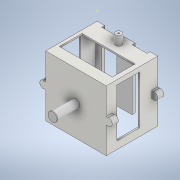
# Autodesk Inventor part: elevador_caixa_com_estabi v2
Saved by Autodesk Inventor 2021 (Build 250183000, 183)
## iProperties
Created: 2020-09-22
Part Number: elevador_caixa_com_estabi v2
Material: Genérico
Document SubType Name: Modeling
Designer: evert
Density: 1 g/cm^3
Appearance: Padrão
Author: evert
Autodesk Inventor part; units mm, degrees
ref_plane "YZ Plane" through (0, 0, 0) normal (1, 0, 0) x (0, 1, 0)
ref_plane "XZ Plane" through (0, 0, 0) normal (0, 1, 0) x (-1, 0, 0)
ref_plane "XY Plane" through (0, 0, 0) normal (0, 0, 1) x (1, 0, 0)
sketch "Esboço1" plane through (0, 0, 0) normal (0, 0, 1) x (1, 0, 0)
  line L0 (0, 0) -> (40, 0)
  line L1 (40, 0) -> (40, 40)
  line L2 (40, 40) -> (0, 40)
  line L3 (0, 40) -> (0, 0)
  dimension "d0" = 40
  dimension "d1" = 40
  constraints: 8 end point, 2 parallel, 1 horizontal, 1 perpendicular
  measures "d0" distance of L2.end L1.end
  measures "d1" distance of L0.end L1.end
extrude "Extrusão1" add sketch "Esboço1" along normal blind 2
sketch "Esboço2" plane through (0, 0, 2) normal (0, 0, 1) x (1, 0, 0)
  line L0 (0, 40) -> (0, 0) projected
  line L1 (0, 0) -> (1, 0)
  line L2 (0, 0) -> (40, 0) projected
  line L3 (0, 0) -> (0, 40)
  line L4 (40, 40) -> (0, 40) projected
  line L5 (40, 0) -> (40, 40) projected
  line L6 (40, 40) -> (40, 0)
  line L7 (40, 0) -> (39, 0)
  line L8 (39, 0) -> (39, 39)
  line L9 (39, 39) -> (1, 39)
  line L10 (1, 39) -> (1, 0)
  constraints: 14 end point, 2 collinear, 2 perpendicular, 2 point on line, 1 vertical
extrude "Extrusão2" add sketch "Esboço2" along normal blind 10 contours L4 L5 L2 L8 L9 L10 L1 L0
sketch "Esboço3" plane through (0, 0, 12) normal (0, 0, 1) x (1, 0, 0)
  line L0 (0, 40) -> (2, 40)
  line L1 (40, 40) -> (0, 40) projected
  line L2 (1, 39) -> (39, 39) projected
  line L3 (2, 39) -> (1, 39)
  line L4 (1, 39) -> (1, 38)
  line L5 (1, 0) -> (1, 39) projected
  line L6 (0, 38) -> (0, 40)
  line L7 (2, 40) -> (2, 39)
  line L8 (1, 38) -> (0, 38)
  line L9 (0, 40) -> (0, 0) projected
  constraints: 12 end point, 3 point on line, 1 collinear, 1 parallel, 1 perpendicular, 1 vertical
extrude "Extrusão3" add sketch "Esboço3" along normal blind 20
sketch "Esboço4" plane through (0, 0, 12) normal (0, 0, 1) x (1, 0, 0)
  line L0 (40, 40) -> (37, 40)
  line L1 (40, 40) -> (0, 40) projected
  line L2 (39, 39) -> (1, 39) projected
  line L3 (37, 39) -> (39, 39)
  line L4 (39, 39) -> (39, 37)
  line L5 (39, 39) -> (39, 0) projected
  line L6 (40, 0) -> (40, 40) projected
  line L7 (40, 37) -> (40, 40)
  line L8 (37, 40) -> (37, 39)
  line L9 (39, 37) -> (40, 37)
  line L10 (40, 40) -> (37, 40)
  line L11 (37, 39) -> (39, 39)
  line L12 (39, 39) -> (39, 37)
  point P0 (0, 0)
  constraints: 18 end point, 3 collinear, 2 horizontal, 2 perpendicular, 2 point on line
extrude "Extrusão4" add sketch "Esboço4" along normal blind 20
sketch "Esboço5" plane through (0, 0, 2) normal (0, 0, 1) x (1, 0, 0)
  point P0 (0, 0)
sketch "Esboço6" plane through (0, 0, 12) normal (0, 0, 1) x (1, 0, 0)
  line L0 (0, 38) -> (0, 0) projected
  line L1 (1, 0) -> (1, 38) projected
  line L2 (0, 0) -> (1, 0)
  line L3 (1, 0) -> (1, 5)
  line L4 (1, 5) -> (0, 5)
  line L5 (0, 5) -> (0, 0)
  line L6 (0, 0) -> (40, 0) projected
  line L7 (39, 0) -> (39, 39) projected
  line L8 (40, 0) -> (39, 0)
  line L9 (39, 0) -> (39, 5)
  line L10 (39, 5) -> (40, 5)
  line L11 (40, 5) -> (40, 0)
  constraints: 16 end point, 4 parallel, 3 point on line, 2 horizontal, 2 perpendicular
extrude "Extrusão5" add sketch "Esboço6" along normal blind 20
sketch "Esboço7" plane through (0, 0, 32) normal (0, 0, 1) x (1, 0, 0)
  line L0 (0, 38) -> (0, 5) projected
  line L1 (0, 38) -> (1, 38)
  line L2 (1, 5) -> (1, 38) projected
  line L3 (1, 38) -> (1, 5)
  line L4 (1, 5) -> (0, 5)
  line L5 (0, 40) -> (0, 38) projected
  line L6 (0, 5) -> (0, 38)
  point P0 (0, 0)
  constraints: 8 end point, 2 perpendicular, 1 collinear, 1 horizontal
extrude "Extrusão6" add sketch "Esboço7" against normal blind 5
sketch "Esboço8" plane through (0, 0, 32) normal (0, 0, 1) x (1, 0, 0)
  line L0 (2, 40) -> (0, 40) projected
  line L1 (39, 39) -> (1, 39) projected
  line L2 (2, 40) -> (37, 40)
  line L3 (37, 40) -> (37, 39)
  line L4 (37, 39) -> (2, 39)
  line L5 (2, 39) -> (2, 40)
  point P0 (0, 0)
  constraints: 8 end point, 2 parallel, 1 horizontal, 1 perpendicular, 1 point on line
extrude "Extrusão7" add sketch "Esboço8" against normal blind 5
sketch "Esboço9" plane through (0, 0, 32) normal (0, 0, 1) x (1, 0, 0)
  line L0 (40, 0) -> (40, 40) projected
  line L1 (39, 37) -> (40, 37)
  line L2 (40, 37) -> (40, 5)
  line L3 (40, 5) -> (39, 5)
  line L4 (39, 5) -> (39, 37)
  point P0 (0, 0)
  constraints: 8 end point, 2 parallel, 1 horizontal, 1 perpendicular, 1 point on line
extrude "Extrusão8" add sketch "Esboço9" against normal blind 5
sketch "Esboço10" plane through (0, 0, 32) normal (0, 0, 1) x (1, 0, 0)
  line L0 (40, 40) -> (0, 40) projected
  line L1 (0, 40) -> (0, 0) projected
  line L2 (40, 40) -> (0, 40)
  line L3 (0, 40) -> (0, 0)
  line L4 (0, 0) -> (40, 0)
  line L5 (40, 0) -> (40, 40)
  constraints: 8 end point, 2 parallel, 1 horizontal, 1 perpendicular
extrude "Extrusão9" add sketch "Esboço10" along normal blind 2
sketch "Esboço11" plane through (0, 40, 0) normal (0, 1, 0) x (1, 0, 0)
  line L0 (40, 0) -> (0, 0) projected
  line L1 (20, 0) -> (20, -12)
  line L2 (2, -12) -> (37, -12) projected
  line L3 (40, -5.8482) -> (0, -5.8482)
  circle A0 centre (20, -5.8482) radius 2
  dimension "d20" = 4
  constraints: 4 end point, 2 midpoint, 1 centre point, 1 horizontal, 1 point on line, 1 vertical
  measures "d20" diameter of A0
extrude "Extrusão10" add sketch "Esboço11" along normal blind 6
sketch "Esboço12" plane through (20, 46, 5.8482) normal (0, 1, 0) x (1, 0, 0)
  point P0 (-20, 5.8482)
sketch "Esboço13" plane through (20, 46, 5.8482) normal (0, 1, 0) x (1, 0, 0)
  point P0 (-20, 5.8482)
  point P1 (0.0054, -0.0097)
hole "Furo1" at (20.0054, 46, 5.8579) direction (0, -1, 0) diameter 1.0109 depth 3.799 thread size "00-90 NS" class "2B" standard "ANSI Unified Screw Threads"
sketch "Esboço14" plane through (0, 0, 34) normal (0, 0, 1) x (1, 0, 0)
  line L0 (0, 40) -> (0, 0) projected
  line L1 (0, 40) -> (0, 20)
  circle A0 centre (-1.4378, 20) radius 2.5
  line L2 (-1.4378, 17.5) -> (-0.8668, 18) construction
  line L3 (-0.8668, 18) -> (0, 17.5) construction
  spline S0 degree 2 poles (-1.4378, 17.5) (-0.8668, 18) (0, 17.5) knots 1 1 1 2 2 2
  line L4 (40, 0) -> (40, 40) projected
  line L5 (40, 40) -> (40, 0)
  line L6 (40, 40) -> (0, 40) projected
  line L7 (0, 40) -> (0, 0)
  circle A1 centre (41.4279, 20) radius 2.5
  line L8 (41.4279, 17.5) -> (40.8569, 18) construction
  line L9 (40.8569, 18) -> (39.9901, 17.5) construction
  spline S1 degree 2 poles (41.4279, 17.5) (40.8569, 18) (39.9901, 17.5) knots 1 1 1 2 2 2
  line L10 (-1.4378, 20) -> (40, 20)
  line L11 (-1.4378, 22.5) -> (-0.8668, 22) construction
  line L12 (-0.8668, 22) -> (0, 22.5) construction
  spline S2 degree 2 poles (-1.4378, 22.5) (-0.8668, 22) (0, 22.5) knots 1 1 1 2 2 2
  spline S3 degree 2 poles (41.4279, 22.5) (40.8569, 22) (39.9901, 22.5) knots 1 1 1 2 2 2
  line L13 (41.4279, 22.5) -> (40.8569, 22) construction
  line L14 (40.8569, 22) -> (39.9901, 22.5) construction
  point P0 (40, 22.4943)
  point P1 (40, 17.5057)
  point P2 (0, 22.5)
  dimension "d30" = 5
  constraints: 8 end point, 6 symmetric about line, 2 collinear, 2 midpoint, 1 point on line, 18 other
extrude "Extrusão11" add sketch "Esboço14" against normal blind 4 contours L0 A0 S2 | L0 A0 S0 S2 | S3 A1 L4 | A1 S3 S1 L4 | L0 S0 A0 | A1 S1 L4
sketch "Esboço15" plane through (0, 0, 0) normal (0, 0, -1) x (-1, 0, 0)
  spline S0 degree 2 poles (1.4304, 17.5) (0.8594, 18) (-0.0074, 17.5) knots 1 1 1 2 2 2
  line L0 (1.4304, 17.5) -> (0.8594, 18) construction
  line L1 (0.8594, 18) -> (-0.0074, 17.5) construction
  circle A0 centre (1.4304, 20) radius 2.5
  spline S1 degree 2 poles (1.4304, 22.5) (0.8594, 22) (-0.0074, 22.5) knots 1 1 1 2 2 2
  line L2 (1.4304, 22.5) -> (0.8594, 22) construction
  line L3 (0.8594, 22) -> (-0.0074, 22.5) construction
  line L4 (-40, 40) -> (0, 40) projected
  line L5 (-40, 40) -> (-40, 0)
  line L6 (-39, 0) -> (-39, 39) projected
  spline S2 degree 2 poles (-41.4206, 17.5) (-40.8496, 18) (-39.9828, 17.5) knots 1 1 1 2 2 2
  line L7 (-41.4206, 17.5) -> (-40.8496, 18) construction
  line L8 (-40.8496, 18) -> (-39.9828, 17.5) construction
  circle A1 centre (-41.4206, 20) radius 2.5
  spline S3 degree 2 poles (-41.4206, 22.5) (-40.8496, 22) (-39.9828, 22.5) knots 1 1 1 2 2 2
  line L9 (-41.4206, 22.5) -> (-40.8496, 22) construction
  line L10 (-40.8496, 22) -> (-39.9828, 22.5) construction
  line L11 (0, 40) -> (0, 0) projected
  line L12 (0, 17.9497) -> (0, 22.0503)
  line L13 (-40, 0) -> (-40, 40) projected
  line L14 (-40, 17.9428) -> (-40, 22.0572)
  line L15 (-40, 17.9428) -> (-40, 22.0572)
  point P0 (1.4378, 22.5)
  point P1 (0, 17.5043)
  point P2 (0, 22.4957)
  point P3 (-40, 17.5099)
  point P4 (-40, 22.4901)
  constraints: 8 end point, 6 point on circle, 4 point on line, 2 centre point, 1 collinear, 1 parallel, 12 other
extrude "Extrusão12" add sketch "Esboço15" against normal blind 4 contours S0 A0 L11 S1 | S0 L11 A0 | L11 S1 A0 | A1 S3 L5 | L5 A1 S2 S3 | L5 S2 A1
sketch "Esboço16" plane through (40, 40, 34) normal (1, 0, 0) x (0, 0, -1)
  point P0 (34, -40)
sketch "Esboço17" plane through (0, 0, 34) normal (0, 0, 1) x (1, 0, 0)
  line L0 (39, 37) -> (39, 5) projected
  line L1 (39, 20) -> (1, 20)
  line L2 (1, 5) -> (1, 38) projected
  line L3 (0, 0) -> (40, 0) projected
  line L4 (40, 0) -> (0, 0)
  line L5 (0, 0) -> (20, 0)
  line L6 (20, 40) -> (20, 0)
  circle A0 centre (20, 20) radius 2.5
  dimension "d36" = 5
  constraints: 8 end point, 2 midpoint, 2 point on line, 1 centre point, 1 collinear, 1 horizontal, 1 perpendicular
  measures "d36" diameter of A0
extrude "Extrusão13" add sketch "Esboço17" along normal blind 15
sketch "Esboço18" plane through (20, 20, 49) normal (0, 0, 1) x (1, 0, 0)
  circle A0 centre (0, 0) radius 2.5 projected
  circle A1 centre (0, 0) radius 3
  point P0 (-20, -20)
  dimension "d39" = 6
  constraints: 1 centre point, 1 coincident
  measures "d39" diameter of A1
extrude "Extrusão14" add sketch "Esboço18" along normal blind 0.5 contours A0 | A1
sketch "Esboço20" plane through (0, 0, 2) normal (0, 0, 1) x (1, 0, 0)
  line L0 (0, 0) -> (40, 0) projected
  line L1 (0, 0) -> (10, 0)
  line L2 (10, 40) -> (0, 40)
  line L3 (0, 40) -> (0, 0)
  line L4 (40, 40) -> (0, 40) projected
  line L5 (25, 0) -> (35, 0)
  line L6 (35, 0) -> (35, 40)
  line L7 (35, 40) -> (25, 40)
  line L8 (25, 40) -> (25, 0)
  line L9 (1, 0) -> (39, 0) projected
  line L10 (5, 0) -> (15, 0)
  line L11 (15, 0) -> (15, 40)
  line L12 (15, 40) -> (5, 40)
  line L13 (5, 40) -> (5, 0)
  dimension "d44" = 10
  dimension "d45" = 10
  dimension "d46" = 40
  constraints: 22 end point, 5 parallel, 4 point on line, 3 horizontal, 2 perpendicular
  measures "d44" distance of L7.end L6.end
  measures "d45" distance of L12.end L11.end
  measures "d46" distance of L11.end L10.end
extrude "Extrusão15" cut sketch "Esboço20" against normal blind 10 contours L13 L2 L4 L11 L0 | L8 L4 L6 L0
